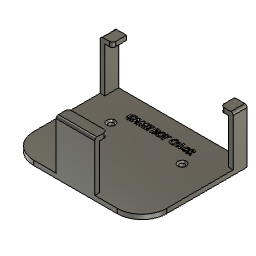
Nintendo Game Boy Color (Autodesk Fusion 360 design; units mm, degrees)
Autodesk Fusion 360 part; units mm, degrees
sketch "Sketch1" plane through (0, 0, 0) normal (0, 0, 1) x (1, 0, 0)
  line L0 (0, 0) -> (-86, 0)
  line L1 (-86, 0) -> (-86, 68)
  line L2 (-86, 68) -> (0, 68)
  line L3 (0, 68) -> (0, 0)
  dimension "d1" = 86
  dimension "d2" = 68
  constraint horizontal L0
  constraint vertical L1
  constraint horizontal L2
  constraint vertical L3
  constraint coincident L0.start L3.end
  measures "d1" distance of L0.start L0.end
  measures "d2" distance of L0.start L2.end
extrude "Extrude1" add sketch "Sketch1" along normal blind 35
sketch "Sketch2" plane through (0, 0, 35) normal (0, 0, 1) x (-1, 0, 0)
  line L0 (0, -68) -> (86, -68)
  line L1 (86, -68) -> (86, 0)
  line L2 (86, 0) -> (0, 0)
  line L3 (0, 0) -> (0, -68)
  line L4 (86, -68) -> (78, -68)
  line L5 (78, -68) -> (78, -59)
  line L6 (78, -59) -> (86, -59)
  line L7 (86, -59) -> (86, -68)
  line L8 (0, -68) -> (8, -68)
  line L9 (8, -68) -> (8, -59)
  line L10 (8, -59) -> (0, -59)
  line L11 (0, -59) -> (0, -68)
  line L12 (43, 0) -> (30.5, 0)
  line L13 (30.5, 0) -> (30.5, -8)
  line L14 (30.5, -8) -> (43, -8)
  line L15 (43, -8) -> (43, 0)
  line L16 (43, 0) -> (55.5, 0)
  line L17 (55.5, 0) -> (55.5, -8)
  line L18 (55.5, -8) -> (43, -8)
  line L19 (43, -8) -> (43, 0)
  dimension "d5" = 8
  dimension "d6" = 9
  dimension "d7" = 8
  dimension "d8" = 9
  dimension "d9" = 12.5
  dimension "d10" = 8
  dimension "d11" = 12.5
  dimension "d12" = 8
  constraint horizontal L4
  constraint vertical L5
  constraint horizontal L6
  constraint vertical L7
  constraint coincident L0.end L1.start
  constraint horizontal L8
  constraint vertical L9
  constraint horizontal L10
  constraint vertical L11
  constraint coincident L0.start L3.end
  constraint horizontal L12
  constraint vertical L13
  constraint horizontal L14
  constraint vertical L15
  constraint midpoint L2 L12.start
  constraint horizontal L16
  constraint vertical L17
  constraint horizontal L18
  constraint vertical L19
  measures "d5" distance of L0.end L4.end
  measures "d6" distance of L0.end L6.end
  measures "d7" distance of L0.start L8.end
  measures "d8" distance of L0.start L10.end
  measures "d9" distance of L12.start L12.end
  measures "d10" distance of L12.start L14.end
  measures "d11" distance of L12.start L16.end
  measures "d12" distance of L12.start L14.end
extrude "Extrude2" cut sketch "Sketch2" against normal blind 32 contours L0 L1 L2 L3 L5 L6 L9 L10 L13 L14 L17 L18
sketch "Sketch3" plane through (0, 59, 0) normal (0, -1, 0) x (1, 0, 0)
  line L0 (-78, 35) -> (-86, 35)
  line L1 (-86, 35) -> (-86, 3)
  line L2 (-86, 3) -> (-78, 3)
  line L3 (-78, 3) -> (-78, 35)
  line L4 (-78, 3) -> (-83, 3)
  line L5 (-83, 3) -> (-83, 32)
  line L6 (-83, 32) -> (-78, 32)
  line L7 (-78, 32) -> (-78, 3)
  dimension "d15" = 5
  dimension "d16" = 29
  constraint horizontal L4
  constraint vertical L5
  constraint horizontal L6
  constraint vertical L7
  constraint coincident L2.end L3.start
  measures "d15" distance of L2.end L4.end
  measures "d16" distance of L2.end L6.end
extrude "Extrude3" cut sketch "Sketch3" against normal blind 9 contours L2 L3 L4 L5 L6 L7
sketch "Sketch4" plane through (0, 59, 0) normal (0, -1, 0) x (1, 0, 0)
  line L0 (0, 35) -> (-8, 35)
  line L1 (-8, 35) -> (-8, 3)
  line L2 (-8, 3) -> (0, 3)
  line L3 (0, 3) -> (0, 35)
  line L4 (-8, 3) -> (-3, 3)
  line L5 (-3, 3) -> (-3, 32)
  line L6 (-3, 32) -> (-8, 32)
  line L7 (-8, 32) -> (-8, 3)
  dimension "d19" = 5
  dimension "d20" = 29
  constraint horizontal L4
  constraint vertical L5
  constraint horizontal L6
  constraint vertical L7
  constraint coincident L1.end L2.start
  measures "d19" distance of L1.end L4.end
  measures "d20" distance of L1.end L6.end
extrude "Extrude4" cut sketch "Sketch4" against normal blind 9 contours L1 L2 L4 L5 L6 L7
sketch "Sketch5" plane through (-30.5, 0, 0) normal (1, 0, 0) x (0, 1, 0)
  line L0 (8, 35) -> (0, 35)
  line L1 (0, 35) -> (0, 3)
  line L2 (0, 3) -> (8, 3)
  line L3 (8, 3) -> (8, 35)
  line L4 (8, 3) -> (3, 3)
  line L5 (3, 3) -> (3, 32)
  line L6 (3, 32) -> (8, 32)
  line L7 (8, 32) -> (8, 3)
  dimension "d23" = 5
  dimension "d24" = 29
  constraint horizontal L4
  constraint vertical L5
  constraint horizontal L6
  constraint vertical L7
  constraint coincident L2.end L3.start
  measures "d23" distance of L2.end L4.end
  measures "d24" distance of L2.end L6.end
extrude "Extrude5" cut sketch "Sketch5" against normal blind 25 contours L2 L3 L4 L5 L6 L7
fillet "Fillet1" radius 16 2 edges at (0, 0, 1.5) (-86, 0, 1.5)
fillet "Fillet2" radius 2 2 edges at (-78, 59, 33.5) (-8, 59, 33.5)
fillet "Fillet3" radius 2 2 edges at (-30.5, 8, 33.5) (-55.5, 8, 33.5)
sketch "Logo" plane through (0, 0, 3) normal (0, 0, 1) x (1, 0, 0)
  line L0 (-60.5665, 56.7778) -> (-60.4098, 57.7813)
  line L1 (-60.4098, 57.7813) -> (-61.8278, 57.7813)
  spline S0 degree 3 poles (-61.8278, 57.7813) (-61.8279, 57.7813) (-64.2375, 57.7468) (-64.4374, 55.2333) knots 2 2 2 2 3 3 3 3
  spline S1 degree 3 poles (-64.4374, 55.2333) (-64.4374, 55.2332) (-64.6727, 53.2517) (-62.524, 53.0287) knots 3 3 3 3 4 4 4 4
  spline S2 degree 3 poles (-62.524, 53.0287) (-62.5239, 53.0287) (-60.6711, 52.8057) (-60.5926, 55.3532) knots 4 4 4 4 5 5 5 5
  line L2 (-60.5926, 55.3532) -> (-62.402, 55.3532)
  line L3 (-62.402, 55.3532) -> (-62.4803, 54.5304)
  line L4 (-62.4803, 54.5304) -> (-61.7407, 54.5304)
  spline S3 degree 3 poles (-61.7407, 54.5304) (-61.7407, 54.5304) (-61.932, 54.058) (-62.4458, 54.058) (-62.9587, 54.058) (-63.3762, 54.6414) (-63.3415, 55.2077) knots 8 8 8 8 9 9 9 10 10 10 10
  spline S4 degree 3 poles (-63.3415, 55.2077) (-63.307, 55.7741) (-63.1066, 56.6316) (-61.906, 56.7862) knots 10 10 10 10 11 11 11 11
  spline S5 degree 3 poles (-61.906, 56.7862) (-61.906, 56.7778) (-60.5665, 56.7778) (-60.5665, 56.7778) knots 11 11 11 11 12 12 12 12
  line L5 (-59.1844, 55.4138) -> (-58.8709, 56.1942)
  line L6 (-58.8709, 56.1942) -> (-58.6537, 55.4047)
  line L7 (-58.6537, 55.4047) -> (-59.1844, 55.4138)
  line L8 (-52.7472, 57.6616) -> (-53.7387, 57.6616)
  line L9 (-53.7387, 57.6616) -> (-54.8081, 55.6368)
  line L10 (-54.8081, 55.6368) -> (-55.2872, 57.6698)
  line L11 (-55.2872, 57.6698) -> (-56.2701, 57.6698)
  line L12 (-56.2701, 57.6698) -> (-57.4008, 54.1008)
  line L13 (-57.4008, 54.1008) -> (-58.1043, 57.627)
  line L14 (-58.1043, 57.627) -> (-59.1314, 57.627)
  line L15 (-59.1314, 57.627) -> (-61.1233, 53.2428)
  line L16 (-61.1233, 53.2428) -> (-59.993, 53.2344)
  line L17 (-59.993, 53.2344) -> (-59.4713, 54.4865)
  line L18 (-59.4713, 54.4865) -> (-58.5663, 54.4865)
  line L19 (-58.5663, 54.4865) -> (-58.2619, 53.2517)
  line L20 (-58.2619, 53.2517) -> (-56.5311, 53.2517)
  line L21 (-56.5311, 53.2517) -> (-55.8611, 55.7825)
  line L22 (-55.8611, 55.7825) -> (-55.3397, 53.2857)
  line L23 (-55.3397, 53.2857) -> (-54.7825, 53.2857)
  line L24 (-54.7825, 53.2857) -> (-53.6428, 55.7998)
  line L25 (-53.6428, 55.7998) -> (-53.5384, 53.2428)
  line L26 (-53.5384, 53.2428) -> (-52.5209, 53.2428)
  line L27 (-52.5209, 53.2428) -> (-52.7472, 57.6616)
  line L28 (-51.1469, 56.0397) -> (-49.7556, 56.0397)
  line L29 (-52.4169, 53.2517) -> (-51.8611, 57.73)
  line L30 (-51.0519, 56.6662) -> (-51.1469, 56.0397)
  line L31 (-51.3567, 54.3325) -> (-49.7821, 54.3325)
  line L32 (-49.9733, 53.2517) -> (-52.4169, 53.2517)
  line L33 (-49.4775, 56.6662) -> (-51.0519, 56.6662)
  line L34 (-49.3033, 57.73) -> (-49.4775, 56.6662)
  line L35 (-49.7556, 56.0397) -> (-49.9208, 55.0277)
  line L36 (-51.2518, 55.0277) -> (-51.3567, 54.3325)
  line L37 (-49.7821, 54.3325) -> (-49.9733, 53.2517)
  line L38 (-51.8611, 57.73) -> (-49.3033, 57.73)
  line L39 (-49.9208, 55.0277) -> (-51.2518, 55.0277)
  line L40 (-46.5634, 55.8768) -> (-47.1811, 55.8598)
  line L41 (-47.1811, 55.8598) -> (-47.034, 56.7007)
  line L42 (-47.034, 56.7007) -> (-46.4597, 56.7007)
  spline S6 degree 3 poles (-46.4597, 56.7007) (-46.4597, 56.7007) (-46.0769, 56.6143) (-46.0769, 56.3487) knots 3 3 3 3 4 4 4 4
  spline S7 degree 3 poles (-46.0769, 56.3487) (-46.0588, 55.9799) (-46.5633, 55.8768) (-46.5634, 55.8768) knots 4 4 4 4 5 5 5 5
  line L43 (-46.5902, 54.1008) -> (-47.4686, 54.0923)
  line L44 (-47.4686, 54.0923) -> (-47.3125, 54.9844)
  line L45 (-47.3125, 54.9844) -> (-46.5114, 54.9844)
  spline S8 degree 3 poles (-46.5114, 54.9844) (-46.5114, 54.9844) (-46.1116, 54.8819) (-46.1201, 54.5386) knots 3 3 3 3 4 4 4 4
  spline S9 degree 3 poles (-46.1201, 54.5386) (-46.1289, 54.1956) (-46.5902, 54.1008) (-46.5902, 54.1008) knots 4 4 4 4 5 5 5 5
  spline S10 degree 3 poles (-45.0586, 56.5031) (-44.9456, 57.6527) (-46.0588, 57.7645) (-46.0588, 57.7645) knots 0 0 0 0 1 1 1 1
  line L46 (-46.0588, 57.7645) -> (-47.7993, 57.7645)
  line L47 (-47.7993, 57.7645) -> (-48.5301, 53.2607)
  spline S11 degree 3 poles (-48.5301, 53.2607) (-48.53, 53.2607) (-46.4159, 53.2685) (-46.4247, 53.2607) knots 3 3 3 3 4 4 4 4
  spline S12 degree 3 poles (-46.4247, 53.2607) (-45.5286, 53.3887) (-45.2414, 53.9035) (-45.1715, 54.5734) knots 4 4 4 4 5 5 5 5
  spline S13 degree 3 poles (-45.1715, 54.5734) (-45.1024, 55.2417) (-45.5723, 55.5249) (-45.5724, 55.525) knots 5 5 5 5 6 6 6 6
  spline S14 degree 3 poles (-45.5724, 55.525) (-45.5723, 55.525) (-45.1634, 55.6971) (-45.0586, 56.5031) knots 6 6 6 6 7 7 7 7
  spline S15 degree 3 poles (-43.2966, 54.1156) (-43.2967, 54.1156) (-44.2401, 54.102) (-44.181, 55.388) (-44.1219, 56.6749) (-43.0604, 56.7549) (-43.0531, 56.7624) knots 0 0 0 0 1 1 1 2 2 2 2
  spline S16 degree 3 poles (-43.0531, 56.7624) (-43.0604, 56.7549) (-42.331, 56.8132) (-42.1688, 55.6208) knots 2 2 2 2 3 3 3 3
  spline S17 degree 3 poles (-42.1688, 55.6208) (-42.2053, 54.0211) (-43.2966, 54.1156) (-43.2966, 54.1156) knots 3 3 3 3 4 4 4 4
  spline S18 degree 3 poles (-42.9058, 57.7006) (-44.9178, 57.4749) (-45.0879, 55.41) (-45.0879, 55.41) knots 0 0 0 0 1 1 1 1
  spline S19 degree 3 poles (-45.0879, 55.41) (-45.0879, 55.4099) (-45.3305, 53.345) (-43.3481, 53.2213) knots 1 1 1 1 2 2 2 2
  spline S20 degree 3 poles (-43.3481, 53.2213) (-41.0994, 53.272) (-41.2027, 55.7149) (-41.2027, 55.715) knots 2 2 2 2 3 3 3 3
  spline S21 degree 3 poles (-41.2027, 55.715) (-41.2027, 55.715) (-41.0403, 57.6857) (-42.9058, 57.7006) knots 3 3 3 3 4 4 4 4
  line L48 (-39.8756, 53.2213) -> (-39.6179, 55.4026)
  line L49 (-38.0478, 57.6929) -> (-39.1531, 57.6929)
  line L50 (-40.4659, 57.7006) -> (-41.5491, 57.7078)
  line L51 (-39.1531, 57.6929) -> (-40.0451, 56.3043)
  line L52 (-41.5491, 57.7078) -> (-40.606, 55.5193)
  line L53 (-39.6179, 55.4026) -> (-38.0478, 57.6929)
  line L54 (-40.9152, 53.2213) -> (-39.8756, 53.2213)
  line L55 (-40.606, 55.5193) -> (-40.9152, 53.2213)
  line L56 (-40.0451, 56.3043) -> (-40.4659, 57.7006)
  spline S22 degree 3 poles (-33.5021, 57.1849) (-33.6541, 57.9905) (-34.4911, 57.9995) (-35.1244, 57.7868) knots 0 0 0 0 1 1 1 1
  spline S23 degree 3 poles (-35.1244, 57.7868) (-35.9789, 57.4993) (-36.4101, 56.8443) (-36.7138, 56.0242) knots 1 1 1 1 2 2 2 2
  spline S24 degree 3 poles (-36.7138, 56.0242) (-37.0103, 55.2221) (-36.8907, 54.2811) (-36.2354, 53.7) knots 2 2 2 2 3 3 3 3
  spline S25 degree 3 poles (-36.2354, 53.7) (-35.6013, 53.138) (-34.6656, 53.1292) (-33.8857, 53.3052) knots 3 3 3 3 4 4 4 4
  spline S26 degree 3 poles (-33.8857, 53.3052) (-33.3079, 53.4349) (-33.5533, 54.3205) (-34.1298, 54.1907) knots 4 4 4 4 5 5 5 5
  spline S27 degree 3 poles (-34.1298, 54.1907) (-35.0668, 53.9794) (-36.1119, 54.2875) (-35.9207, 55.4416) knots 5 5 5 5 6 6 6 6
  spline S28 degree 3 poles (-35.9207, 55.4416) (-35.8513, 55.8639) (-35.6105, 56.4755) (-35.2406, 56.7209) knots 6 6 6 6 7 7 7 7
  spline S29 degree 3 poles (-35.2406, 56.7209) (-35.1022, 56.8123) (-34.4255, 57.1432) (-34.3873, 56.9409) knots 7 7 7 7 8 8 8 8
  spline S30 degree 3 poles (-34.3873, 56.9409) (-34.2779, 56.3594) (-33.3935, 56.6063) (-33.5021, 57.1849) knots 8 8 8 8 9 9 9 9
  spline S31 degree 3 poles (-32.8693, 56.7805) (-33.8329, 56.5212) (-34.1578, 55.4335) (-33.7967, 54.569) knots 0 0 0 0 1 1 1 1
  spline S32 degree 3 poles (-33.7967, 54.569) (-33.3628, 53.5308) (-32.1786, 53.2736) (-31.2549, 53.8613) knots 1 1 1 1 2 2 2 2
  spline S33 degree 3 poles (-31.2549, 53.8613) (-29.4605, 55.0025) (-31.5049, 58.3145) (-33.1219, 56.7277) knots 2 2 2 2 3 3 3 3
  spline S34 degree 3 poles (-33.1219, 56.7277) (-33.5248, 56.3327) (-32.9062, 55.7156) (-32.5045, 56.1104) knots 3 3 3 3 4 4 4 4
  spline S35 degree 3 poles (-32.5045, 56.1104) (-31.8325, 56.7696) (-30.9996, 55.1293) (-31.6957, 54.6153) knots 4 4 4 4 5 5 5 5
  spline S36 degree 3 poles (-31.6957, 54.6153) (-32.8125, 53.791) (-33.6113, 55.6759) (-32.6376, 55.9385) knots 5 5 5 5 6 6 6 6
  spline S37 degree 3 poles (-32.6376, 55.9385) (-32.0941, 56.0845) (-32.3247, 56.9273) (-32.8693, 56.7805) knots 6 6 6 6 7 7 7 7
  spline S38 degree 3 poles (-30.8671, 57.3465) (-30.2975, 56.3201) (-30.3899, 55.0681) (-30.3899, 53.9295) (-30.3899, 53.6563) (-30.1094, 53.4184) (-29.8371, 53.5083) knots 0 0 0 0 1 1 1 2 2 2 2
  spline S39 degree 3 poles (-29.8371, 53.5083) (-29.349, 53.6695) (-28.8463, 53.7517) (-28.3466, 53.8661) knots 2 2 2 2 3 3 3 3
  spline S40 degree 3 poles (-28.3466, 53.8661) (-27.7973, 53.9914) (-28.0302, 54.8334) (-28.5789, 54.7082) knots 3 3 3 3 4 4 4 4
  spline S41 degree 3 poles (-28.5789, 54.7082) (-29.0786, 54.594) (-29.5813, 54.5118) (-30.0694, 54.3505) knots 4 4 4 4 5 5 5 5
  spline S42 degree 3 poles (-30.0694, 54.3505) (-29.885, 54.2099) (-29.7006, 54.0697) (-29.5167, 53.9295) knots 5 5 5 5 6 6 6 6
  spline S43 degree 3 poles (-29.5167, 53.9295) (-29.5167, 55.2415) (-29.4574, 56.6064) (-30.1127, 57.787) knots 6 6 6 6 7 7 7 7
  spline S44 degree 3 poles (-30.1127, 57.787) (-30.386, 58.2797) (-31.1405, 57.839) (-30.8671, 57.3465) knots 7 7 7 7 8 8 8 8
  spline S45 degree 3 poles (-26.6749, 56.3239) (-26.1019, 56.1824) (-25.7176, 55.7152) (-25.8562, 55.11) knots 0 0 0 0 1 1 1 1
  spline S46 degree 3 poles (-25.8562, 55.11) (-25.9606, 54.6516) (-26.5026, 54.2565) (-26.9692, 54.3857) knots 1 1 1 1 2 2 2 2
  spline S47 degree 3 poles (-26.9692, 54.3857) (-27.2993, 54.4773) (-27.4655, 54.9075) (-27.4876, 55.2111) knots 2 2 2 2 3 3 3 3
  spline S48 degree 3 poles (-27.4876, 55.2111) (-27.5243, 55.7123) (-27.2076, 56.0496) (-26.7476, 56.1872) knots 3 3 3 3 4 4 4 4
  spline S49 degree 3 poles (-26.7476, 56.1872) (-26.1529, 56.3655) (-26.406, 57.2972) (-27.0042, 57.1181) knots 4 4 4 4 5 5 5 5
  spline S50 degree 3 poles (-27.0042, 57.1181) (-27.8851, 56.8542) (-28.4704, 56.1474) (-28.4528, 55.2111) knots 5 5 5 5 6 6 6 6
  spline S51 degree 3 poles (-28.4528, 55.2111) (-28.4371, 54.4178) (-27.9247, 53.6491) (-27.1476, 53.4338) knots 6 6 6 6 7 7 7 7
  spline S52 degree 3 poles (-27.1476, 53.4338) (-26.1743, 53.1638) (-25.202, 53.9711) (-24.9259, 54.8538) knots 7 7 7 7 8 8 8 8
  spline S53 degree 3 poles (-24.9259, 54.8538) (-24.586, 55.9391) (-25.3859, 56.9992) (-26.4182, 57.2546) knots 8 8 8 8 9 9 9 9
  spline S54 degree 3 poles (-26.4182, 57.2546) (-27.0226, 57.4041) (-27.2786, 56.4735) (-26.6749, 56.3239) knots 9 9 9 9 10 10 10 10
  spline S55 degree 3 poles (-22.0713, 53.7641) (-22.5383, 54.2901) (-23.0067, 54.8156) (-23.5022, 55.3147) knots 0 0 0 0 1 1 1 1
  spline S56 degree 3 poles (-23.5022, 55.3147) (-23.8998, 55.7146) (-24.5169, 55.0967) (-24.1197, 54.697) knots 1 1 1 1 2 2 2 2
  spline S57 degree 3 poles (-24.1197, 54.697) (-23.6241, 54.1981) (-23.1565, 53.6726) (-22.6888, 53.1467) knots 2 2 2 2 3 3 3 3
  spline S58 degree 3 poles (-22.6888, 53.1467) (-22.3139, 52.7247) (-21.6982, 53.3449) (-22.0713, 53.7641) knots 3 3 3 3 4 4 4 4
  spline S59 degree 3 poles (-24.1475, 53.3235) (-23.8248, 54.6127) (-23.9973, 55.8885) (-24.0718, 57.1963) knots 0 0 0 0 1 1 1 1
  spline S60 degree 3 poles (-24.0718, 57.1963) (-24.179, 57.0561) (-24.2857, 56.9154) (-24.3925, 56.7751) knots 1 1 1 1 2 2 2 2
  spline S61 degree 3 poles (-24.3925, 56.7751) (-24.193, 56.82) (-22.9599, 56.9875) (-23.1736, 56.4857) knots 2 2 2 2 3 3 3 3
  spline S62 degree 3 poles (-23.1736, 56.4857) (-23.3702, 56.0225) (-23.9786, 55.7027) (-24.3713, 55.4266) knots 3 3 3 3 4 4 4 4
  spline S63 degree 3 poles (-24.3713, 55.4266) (-24.8282, 55.1052) (-24.3925, 54.3473) (-23.9309, 54.6725) knots 4 4 4 4 5 5 5 5
  spline S64 degree 3 poles (-23.9309, 54.6725) (-23.1935, 55.1907) (-22.0588, 55.8618) (-22.3363, 56.9189) knots 5 5 5 5 6 6 6 6
  spline S65 degree 3 poles (-22.3363, 56.9189) (-22.5807, 57.8517) (-23.9127, 57.7783) (-24.6246, 57.6174) knots 6 6 6 6 7 7 7 7
  spline S66 degree 3 poles (-24.6246, 57.6174) (-24.8055, 57.5768) (-24.9557, 57.3818) (-24.9456, 57.1963) knots 7 7 7 7 8 8 8 8
  spline S67 degree 3 poles (-24.9456, 57.1963) (-24.8755, 55.973) (-24.6877, 54.7627) (-24.9894, 53.5553) knots 8 8 8 8 9 9 9 9
  spline S68 degree 3 poles (-24.9894, 53.5553) (-25.1262, 53.0089) (-24.2841, 52.7772) (-24.1475, 53.3235) knots 9 9 9 9 10 10 10 10
extrude "Extrude6" cut sketch "Logo" against normal blind 2 contours L0 L1 S0 S1 S2 L2 L3 L4 S3 S4 S5 | L8 L9 L10 L11 L12 L13 L14 L15 L16 L17 L18 L19 L20 L21 L22 L23 L24 L25 L26 L27 | L28 L29 L30 L31 L32 L33 L34 L35 L36 L37 L38 L39 | S10 L46 L47 S11 S12 S13 S14 | S18 S19 S20 S21 | L48 L49 L50 L51 L52 L53 L54 L55 L56 | S22 S23 S24 S25 S26 S27 S28 S29 S30 | S31 S34 S35 S37 | S31 S32 S33 S34 | S41 S42 S43 | S38 S39 S40 S41 S43 S44 S51 | S40 S51 | S45 S49 S54 | S40 S49 S50 S51 S52 S53 S54 | S55 S57 S58 S59 S63 S64 | S55 S56 S59 S63 S64 | S59 S60 S61 | S55 S56 S57 S59 S62 S63 S64 S65 S66 S67 S68 | S57 S59 S63 | S56 S57 S59 S63 | S56 S57 S59 S62 S63
hole "Hole1" at (-66, 46, 3) direction (0, 0, -1) diameter 3.5 depth 3 tip angle 118 countersink diameter 5.5 countersink angle 90
hole "Hole2" at (-20, 46, 3) direction (0, 0, -1) diameter 3.5 depth 3 tip angle 118 countersink diameter 5.5 countersink angle 90
fillet "Fillet4" radius 1.5 3 edges at (-43, 0, 35) (-86, 63.5, 35) (0, 63.5, 35)
